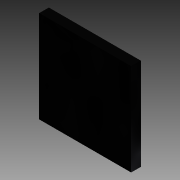
# Autodesk Inventor part: PIC16Chip
Saved by Autodesk Inventor 2014 (Build 180170000, 170)
## iProperties
Created: 2015-03-25
Part Number: PIC16Chip
Material: Generic
Document SubType Name: Modeling
Designer: Owner
Density: 1 g/cm^3
Appearance: Black
Author: Owner
Autodesk Inventor part; units mm, degrees
ref_plane "YZ Plane" through (0, 0, 0) normal (1, 0, 0) x (0, 1, 0)
ref_plane "XZ Plane" through (0, 0, 0) normal (0, 1, 0) x (-1, 0, 0)
ref_plane "XY Plane" through (0, 0, 0) normal (0, 0, 1) x (1, 0, 0)
sketch "Sketch1" plane through (0, 0, 0) normal (0, 0, 1) x (1, 0, 0)
  line L0 (-5.1519, 3.0105) -> (6.2481, 3.0105)
  line L1 (6.2481, 3.0105) -> (6.2481, -8.3895)
  line L2 (6.2481, -8.3895) -> (-5.1519, -8.3895)
  line L3 (-5.1519, -8.3895) -> (-5.1519, 3.0105)
  point P0 (0, 0)
  dimension "d0" = 11.4
  dimension "d1" = 11.4
  constraints: 8 end point, 2 parallel, 1 horizontal, 1 perpendicular
  measures "d0" distance of L0.start L0.end
  measures "d1" distance of L0.end L1.end
extrude "Extrusion1" add sketch "Sketch1" along normal blind 1.2
body "Solid1"
